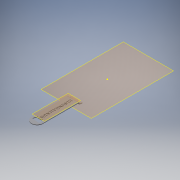
# Autodesk Inventor part: Rost_Heber
Saved by Autodesk Inventor 2018 (Build 220112000, 112)
## iProperties
Created: 2017-10-08
Part Number: Rost_Heber
Material: Generisch
Document SubType Name: Blech
Designer: Jan
Density: 1 g/cm^3
Sheet Metal Rule: Standard_mm
Appearance: Vorgabe
Flat Pattern Width: 4 cm
Flat Pattern Length: 16.3098 cm
Flat Pattern Area: 65.2391 cm^2
Sheet Metal Width: 40,000 mm
Sheet Metal Length: 163,098 mm
Sheet Metal Area: 6523,911 mm^2
Author: Jan
Autodesk Inventor part; units mm, degrees
ref_plane "YZ Plane" through (0, 0, 0) normal (1, 0, 0) x (0, 1, 0)
ref_plane "XZ Plane" through (0, 0, 0) normal (0, 1, 0) x (-1, 0, 0)
ref_plane "XY Plane" through (0, 0, 0) normal (0, 0, 1) x (1, 0, 0)
ref_plane "Arbeitsebene1" through (0, 0, 0) normal (0, 0, 1) x (1, 0, 0)
sketch "Skizze1" plane through (0, 0, 0) normal (0, 0, 1) x (1, 0, 0)
  arc A0 (31.5, -113.5) -> (26.5, -108.5) centre (26.5, -113.5) ccw
  line L0 (26.5, -108.5) -> (-26.5, -108.5)
  arc A1 (-26.5, -108.5) -> (-31.5, -113.5) centre (-26.5, -113.5) ccw
  line L1 (-31.5, -113.5) -> (-31.5, -124.5)
  line L2 (-31.5, -124.5) -> (-71, -124.5)
  arc A2 (-73, -122.5) -> (-71, -124.5) centre (-71, -122.5) ccw
  line L3 (-73, -122.5) -> (-73, 122.5)
  arc A3 (-71, 124.5) -> (-73, 122.5) centre (-71, 122.5) ccw
  line L4 (-71, 124.5) -> (71, 124.5)
  arc A4 (73, 122.5) -> (71, 124.5) centre (71, 122.5) ccw
  line L5 (73, 122.5) -> (73, -122.5)
  arc A5 (71, -124.5) -> (73, -122.5) centre (71, -122.5) ccw
  line L6 (71, -124.5) -> (31.5, -124.5)
  line L7 (31.5, -124.5) -> (31.5, -113.5)
  line L8 (-22.5, -122.5) -> (-22.5, -117.5)
  line L9 (-22.5, -117.5) -> (22.5, -117.5)
  line L10 (22.5, -117.5) -> (22.5, -122.5)
  line L11 (22.5, -122.5) -> (-22.5, -122.5)
  arc A6 (-81, -122.5) -> (-71, -132.5) centre (-71, -122.5) ccw
  line L12 (71, -132.5) -> (-71, -132.5)
  arc A7 (71, -132.5) -> (81, -122.5) centre (71, -122.5) ccw
  line L13 (81, 122.5) -> (81, -122.5)
  arc A8 (81, 122.5) -> (71, 132.5) centre (71, 122.5) ccw
  line L14 (-71, 132.5) -> (71, 132.5)
  arc A9 (-71, 132.5) -> (-81, 122.5) centre (-71, 122.5) ccw
  line L15 (-81, -122.5) -> (-81, 122.5)
  line L16 (-20, -118.5) -> (20, -118.5)
  line L17 (20, -118.5) -> (20, -248.5)
  line L18 (0, -268.5) -> (0, -268.5)
  line L19 (-20, -248.5) -> (-20, -118.5)
  line L20 (-116.2995, 0) -> (116.2995, 0)
  line L21 (0, -314.1009) -> (0, 209.3497)
  arc A10 (-20, -248.5) -> (0, -268.5) centre (0, -248.5) ccw
  arc A11 (0, -268.5) -> (20, -248.5) centre (0, -248.5) ccw
  point P0 (0, 0)
  dimension "HeberBreite" = 40
  dimension "d3" = 1
  dimension "HeberLänge" = 150
  dimension "d5" = 20
  measures "HeberBreite" distance of L16.start L16.end
  measures "d3" distance between parallel lines of L9 L16
  measures "HeberLänge" distance between parallel lines of L18 L16
  measures "d5" radius of A10
extrude "Grobblech1" add sketch "Skizze1" along normal blind 2 contours L21 L11 L19 L16 | L16 L17 L11 L21 | L21 L12 L19 L11 | L11 L17 L12 L21 | L21 A10 L19 L12 | L12 L17 A11 L21
sketch "Skizze2" plane through (20, -120.5, 2) normal (0, 1, 0) x (-1, 0, 0)
  line L0 (40, 0) -> (0, 0)
  line L1 (0, 0) -> (0, -8.05)
  line L2 (0, -8.05) -> (40, -8.05)
  line L3 (40, -8.05) -> (40, 0)
  constraints: 6 end point, 1 horizontal, 1 perpendicular, 1 vertical
edge flange "Lasche1" height 8.05 angle 90 thickness 2 bend radius 2 thickness toward (0, 1, 0) relief straight relief width 2 relief depth 1 edges at (0, -118.5, 0) wall of the first edge with corners at (-20, -120.5, 2) (20, -120.5, 2) (20, -120.5, -6.05) (-20, -120.5, -6.05)
bend "Biegung1"
corner "Ecke1"
sketch "Skizze3" plane through (-20, -120.5, -4.05) normal (0, 0, -1) x (-1, 0, 0)
  line L0 (-40, 0) -> (0, 0)
  line L1 (0, 0) -> (0, 12)
  line L2 (0, 12) -> (-40, 12)
  line L3 (-40, 12) -> (-40, 0)
  constraints: 6 end point, 1 horizontal, 1 perpendicular, 1 vertical
edge flange "Lasche2" height 12 angle 90 thickness 2 bend radius 2 thickness toward (0, 0, -1) relief straight relief width 2 relief depth 1 edges at (0, -118.5, -6.05) wall of the first edge with corners at (20, -120.5, -4.05) (-20, -120.5, -4.05) (-20, -108.5, -4.05) (20, -108.5, -4.05)
bend "Biegung2"
corner "Ecke2"
sketch "Skizze5" plane through (0, 0, 2) normal (0, 0, 1) x (1, 0, 0)
  line L0 (6.947, -239.8347) -> (6.947, -237.7708)
  arc A0 (10.3384, -238.5081) -> (6.947, -237.7708) centre (8.3903, -239.3005) ccw
  line L1 (10.3384, -238.5081) -> (13.6109, -248.7205)
  arc A1 (4.1757, -253.3868) -> (13.6109, -248.7205) centre (7.6304, -248.5) ccw
  line L2 (20, -122.5) -> (-20, -122.5) projected
  line L3 (-20, -248.5) -> (-20, -122.5) projected
  arc A2 (-20, -248.5) -> (20, -248.5) centre (0, -248.5) ccw projected
  line L4 (20, -122.5) -> (20, -248.5) projected
  line L5 (6.947, -239.8347) -> (-0.053, -239.8347)
  line L6 (4.1757, -253.3868) -> (-0.053, -253.3868)
  arc A3 (-7.053, -237.7708) -> (-10.3568, -238.3201) centre (-8.4962, -239.3005) ccw
  line L7 (-10.3568, -238.3201) -> (-13.7136, -248.7954)
  arc A4 (-13.7136, -248.7954) -> (-4.2816, -253.3868) centre (-7.7363, -248.5) ccw
  line L8 (-7.053, -239.8347) -> (-0.053, -239.8347)
  line L9 (-4.2816, -253.3868) -> (-0.053, -253.3868)
  line L10 (-7.053, -237.7708) -> (-7.053, -239.8347)
  line L11 (0, -312.7) -> (0, 206.7)
  dimension "d138" = 0
  constraints: 19 end point, 8 point on circle, 4 centre point, 3 parallel, 2 equal radius, 1 point on line, 1 vertical, 2 other
  measures "d138" vertical distance of A1.centre A2.centre
extrude "Ausklinkung1" cut sketch "Skizze5" against normal blind 2 contours L0 A0 L1 A1 L6 L11 L5 | L11 L6 L9 A4 L7 A3 L10 L8 L5
sketch "Skizze7" plane through (0, 0, 2) normal (0, 0, 1) x (1, 0, 0)
  point P0 (0, 0)
ref_plane "Arbeitsebene2" through (0, 0, 7) normal (0, 0, 1) x (1, 0, 0)
sketch "Skizze8" plane through (0, 0, 7) normal (0, 0, 1) x (1, 0, 0)
  line L0 (4.5218, -125.9558) -> (4.5218, -289.2753) construction
  line L1 (4.5218, -289.2753) -> (-6.6811, -289.2753) construction
  line L2 (-6.6811, -289.2753) -> (-6.6811, -125.9558) construction
  line L3 (-6.6811, -125.9558) -> (4.5218, -125.9558) construction
  line L4 (6.947, -239.8347) -> (6.947, -237.7708) projected
  arc A0 (10.3384, -238.5081) -> (6.947, -237.7708) centre (8.3903, -239.3005) ccw projected
  line L5 (10.3384, -238.5081) -> (13.6109, -248.7205) projected
  arc A1 (4.1757, -253.3868) -> (13.6109, -248.7205) centre (7.6304, -248.5) ccw projected
  line L6 (4.1757, -253.3868) -> (-4.2816, -253.3868) projected
  arc A2 (-13.7136, -248.7954) -> (-4.2816, -253.3868) centre (-7.7363, -248.5) ccw projected
  line L7 (-13.7136, -248.7954) -> (-10.3568, -238.3201) projected
  arc A3 (-7.053, -237.7708) -> (-10.3568, -238.3201) centre (-8.4962, -239.3005) ccw projected
  line L8 (-7.053, -237.7708) -> (-7.053, -239.8347) projected
  line L9 (-7.053, -239.8347) -> (6.947, -239.8347) projected
  line L10 (20, -122.5) -> (-20, -122.5) projected
  line L11 (-20, -248.5) -> (-20, -122.5) projected
  arc A4 (-20, -248.5) -> (20, -248.5) centre (0, -248.5) ccw projected
  line L12 (20, -122.5) -> (20, -248.5) projected
  line L13 (4.3421, -130.9167) -> (-4.6579, -130.9167)
  line L14 (-4.6579, -130.9167) -> (-4.6579, -127.4011)
  line L15 (-4.6579, -127.4011) -> (-4.6579, -127.198)
  spline S0 degree 2 poles (-4.6579, -127.198) (-4.6579, -126.9089) (-4.4782, -126.6042) (-4.3141, -126.6042) knots 0 0 0 1 2 2 2
  spline S1 degree 2 poles (-4.3141, -126.6042) (-4.0485, -126.6042) (-3.9626, -126.9167) knots 0 0 0 1 1 1
  spline S2 degree 2 poles (-3.9626, -126.9167) (-3.8844, -127.1824) (-3.8532, -127.2683) (-3.7907, -127.3152) knots 0 0 0 1 2 2 2
  spline S3 degree 2 poles (-3.7907, -127.3152) (-3.6891, -127.4089) (-3.4548, -127.4089) knots 0 0 0 1 1 1
  line L16 (-3.4548, -127.4089) -> (3.139, -127.4089)
  spline S4 degree 2 poles (3.139, -127.4089) (3.3734, -127.4089) (3.4749, -127.3152) knots 0 0 0 1 1 1
  spline S5 degree 2 poles (3.4749, -127.3152) (3.5374, -127.2683) (3.5687, -127.1824) (3.639, -126.9167) knots 0 0 0 1 2 2 2
  spline S6 degree 2 poles (3.639, -126.9167) (3.7249, -126.6042) (3.9984, -126.6042) knots 0 0 0 1 1 1
  spline S7 degree 2 poles (3.9984, -126.6042) (4.1624, -126.6042) (4.3421, -126.9089) (4.3421, -127.198) knots 0 0 0 1 2 2 2
  line L17 (4.3421, -127.198) -> (4.3421, -127.4011)
  line L18 (4.3421, -127.4011) -> (4.3421, -130.9167)
  line L19 (-4.6579, -131.6355) -> (-3.9469, -131.6355)
  spline S8 degree 2 poles (-3.9469, -131.6355) (-3.8844, -132.1511) (-3.6423, -132.823) (-3.4001, -133.1589) knots 0 0 0 1 2 2 2
  spline S9 degree 2 poles (-3.4001, -133.1589) (-3.1579, -133.5027) (-2.6344, -133.9011) (-2.2048, -134.0886) knots 0 0 0 1 2 2 2
  spline S10 degree 2 poles (-2.2048, -134.0886) (-1.9938, -134.1746) (-1.8454, -134.3621) (-1.8454, -134.5261) knots 0 0 0 1 2 2 2
  spline S11 degree 2 poles (-1.8454, -134.5261) (-1.8454, -134.7527) (-2.0641, -134.9246) (-2.3298, -134.9246) knots 0 0 0 1 2 2 2
  line L20 (-2.3298, -134.9246) -> (-4.6579, -134.9246)
  line L21 (-4.6579, -134.9246) -> (-4.6579, -131.6355)
  line L22 (4.3421, -131.6277) -> (4.3421, -134.8152)
  line L23 (4.3421, -134.8152) -> (2.0062, -134.8152)
  spline S12 degree 2 poles (2.0062, -134.8152) (1.8031, -134.8152) (1.6234, -134.6277) (1.6234, -134.4167) knots 0 0 0 1 2 2 2
  spline S13 degree 2 poles (1.6234, -134.4167) (1.6234, -134.2449) (1.7406, -134.0886) (1.9281, -134.0183) knots 0 0 0 1 2 2 2
  spline S14 degree 2 poles (1.9281, -134.0183) (2.6859, -133.7136) (3.4906, -132.5496) (3.5687, -131.6277) knots 0 0 0 1 2 2 2
  line L24 (3.5687, -131.6277) -> (4.3421, -131.6277)
  line L25 (-0.4626, -131.5886) -> (0.3031, -131.5886)
  spline S15 degree 2 poles (0.3031, -131.5886) (0.4906, -132.0496) (0.9281, -132.4871) (1.2874, -132.5964) knots 0 0 0 1 2 2 2
  spline S16 degree 2 poles (1.2874, -132.5964) (1.5374, -132.6589) (1.7327, -132.8621) (1.7327, -133.0496) knots 0 0 0 1 2 2 2
  spline S17 degree 2 poles (1.7327, -133.0496) (1.7327, -133.3074) (1.5687, -133.4011) knots 0 0 0 1 1 1
  spline S18 degree 2 poles (1.5687, -133.4011) (1.4827, -133.4558) (1.1781, -133.4558) knots 0 0 0 1 1 1
  line L26 (1.1781, -133.4558) -> (-1.3376, -133.4558)
  spline S19 degree 2 poles (-1.3376, -133.4558) (-1.6501, -133.4558) (-1.8844, -133.2917) (-1.8844, -133.0652) knots 0 0 0 1 2 2 2
  spline S20 degree 2 poles (-1.8844, -133.0652) (-1.8844, -132.8855) (-1.6969, -132.6824) (-1.4782, -132.6199) knots 0 0 0 1 2 2 2
  spline S21 degree 2 poles (-1.4782, -132.6199) (-1.0251, -132.4792) (-0.5407, -131.9871) (-0.4626, -131.5886) knots 0 0 0 1 2 2 2
  line L27 (-4.6579, -140.4324) -> (-4.6579, -136.9089)
  line L28 (-4.6579, -136.9089) -> (-4.6579, -136.7058)
  spline S22 degree 2 poles (-4.6579, -136.7058) (-4.6579, -136.4167) (-4.4782, -136.1121) (-4.3141, -136.1121) knots 0 0 0 1 2 2 2
  spline S23 degree 2 poles (-4.3141, -136.1121) (-4.0485, -136.1121) (-3.9626, -136.4246) knots 0 0 0 1 1 1
  spline S24 degree 2 poles (-3.9626, -136.4246) (-3.8844, -136.6902) (-3.8532, -136.7761) (-3.7907, -136.823) knots 0 0 0 1 2 2 2
  spline S25 degree 2 poles (-3.7907, -136.823) (-3.6891, -136.9167) (-3.4548, -136.9167) knots 0 0 0 1 1 1
  line L29 (-3.4548, -136.9167) -> (3.139, -136.9167)
  spline S26 degree 2 poles (3.139, -136.9167) (3.3734, -136.9167) (3.4749, -136.823) knots 0 0 0 1 1 1
  spline S27 degree 2 poles (3.4749, -136.823) (3.5374, -136.7761) (3.5687, -136.6902) (3.639, -136.4246) knots 0 0 0 1 2 2 2
  spline S28 degree 2 poles (3.639, -136.4246) (3.7249, -136.1121) (3.9984, -136.1121) knots 0 0 0 1 1 1
  spline S29 degree 2 poles (3.9984, -136.1121) (4.1624, -136.1121) (4.3421, -136.4167) (4.3421, -136.7058) knots 0 0 0 1 2 2 2
  line L30 (4.3421, -136.7058) -> (4.3421, -136.9089)
  line L31 (4.3421, -136.9089) -> (4.3421, -140.4324)
  line L32 (4.3421, -140.4324) -> (4.3421, -140.6355)
  spline S30 degree 2 poles (4.3421, -140.6355) (4.3421, -140.9246) (4.1624, -141.2292) (3.9984, -141.2292) knots 0 0 0 1 2 2 2
  spline S31 degree 2 poles (3.9984, -141.2292) (3.7249, -141.2292) (3.639, -140.9167) knots 0 0 0 1 1 1
  spline S32 degree 2 poles (3.639, -140.9167) (3.5687, -140.6511) (3.5374, -140.5652) (3.4749, -140.5183) knots 0 0 0 1 2 2 2
  spline S33 degree 2 poles (3.4749, -140.5183) (3.3734, -140.4246) (3.139, -140.4246) knots 0 0 0 1 1 1
  line L33 (3.139, -140.4246) -> (-3.4548, -140.4246)
  spline S34 degree 2 poles (-3.4548, -140.4246) (-3.6891, -140.4246) (-3.7907, -140.5183) knots 0 0 0 1 1 1
  spline S35 degree 2 poles (-3.7907, -140.5183) (-3.8532, -140.5652) (-3.8844, -140.6511) (-3.9626, -140.9167) knots 0 0 0 1 2 2 2
  spline S36 degree 2 poles (-3.9626, -140.9167) (-4.0485, -141.2292) (-4.3141, -141.2292) knots 0 0 0 1 1 1
  spline S37 degree 2 poles (-4.3141, -141.2292) (-4.4782, -141.2292) (-4.6579, -140.9246) (-4.6579, -140.6355) knots 0 0 0 1 2 2 2
  line L34 (-4.6579, -140.6355) -> (-4.6579, -140.4324)
  line L35 (4.5218, -146.1824) -> (3.764, -146.1824)
  spline S38 degree 2 poles (3.764, -146.1824) (3.6468, -145.6902) (3.1781, -145.1746) (2.8421, -145.1746) knots 0 0 0 1 2 2 2
  spline S39 degree 2 poles (2.8421, -145.1746) (2.5062, -145.1746) (2.014, -145.6042) (1.7874, -146.0808) knots 0 0 0 1 2 2 2
  spline S40 degree 2 poles (1.7874, -146.0808) (1.639, -146.4167) (1.2093, -147.5886) knots 0 0 0 1 1 1
  spline S41 degree 2 poles (1.2093, -147.5886) (0.9515, -148.2996) (0.5374, -149.0808) (0.2249, -149.4324) knots 0 0 0 1 2 2 2
  spline S42 degree 2 poles (0.2249, -149.4324) (-0.5876, -150.3621) (-1.7204, -150.3621) knots 0 0 0 1 1 1
  spline S43 degree 2 poles (-1.7204, -150.3621) (-2.5641, -150.3621) (-3.9782, -149.3464) (-4.3844, -148.4636) knots 0 0 0 1 2 2 2
  spline S44 degree 2 poles (-4.3844, -148.4636) (-4.5954, -147.9871) (-4.8376, -146.8621) (-4.8376, -146.3699) knots 0 0 0 1 2 2 2
  line L36 (-4.8376, -146.3699) -> (-4.0876, -146.3699)
  spline S45 degree 2 poles (-4.0876, -146.3699) (-3.9469, -147.0574) (-3.4548, -147.6667) (-3.0329, -147.6667) knots 0 0 0 1 2 2 2
  spline S46 degree 2 poles (-3.0329, -147.6667) (-2.5876, -147.6667) (-2.2516, -147.1902) knots 0 0 0 1 1 1
  spline S47 degree 2 poles (-2.2516, -147.1902) (-2.0329, -146.8777) (-1.7126, -145.9871) knots 0 0 0 1 1 1
  spline S48 degree 2 poles (-1.7126, -145.9871) (-1.3532, -145.0183) (-1.0485, -144.2996) (-0.8454, -143.9636) knots 0 0 0 1 2 2 2
  spline S49 degree 2 poles (-0.8454, -143.9636) (0.0374, -142.4792) (1.5062, -142.4792) knots 0 0 0 1 1 1
  spline S50 degree 2 poles (1.5062, -142.4792) (2.2562, -142.4792) (3.5296, -143.2214) (3.9202, -143.8855) knots 0 0 0 1 2 2 2
  spline S51 degree 2 poles (3.9202, -143.8855) (4.4593, -144.8152) (4.5218, -146.1824) knots 0 0 0 1 1 1
  line L37 (-4.0876, -145.7683) -> (-4.8376, -145.7683)
  spline S52 degree 2 poles (-4.8376, -145.7683) (-4.8376, -145.1199) (-4.5329, -144.3386) knots 0 0 0 1 1 1
  spline S53 degree 2 poles (-4.5329, -144.3386) (-4.4157, -144.0417) (-4.3532, -143.823) (-4.3532, -143.7214) knots 0 0 0 1 2 2 2
  spline S54 degree 2 poles (-4.3532, -143.7214) (-4.3532, -143.5652) (-4.4391, -143.4011) (-4.611, -143.2292) knots 0 0 0 1 2 2 2
  spline S55 degree 2 poles (-4.611, -143.2292) (-4.7516, -143.0886) (-4.7516, -142.9246) knots 0 0 0 1 1 1
  spline S56 degree 2 poles (-4.7516, -142.9246) (-4.7516, -142.4792) (-4.1813, -142.4792) knots 0 0 0 1 1 1
  line L38 (-4.1813, -142.4792) -> (-1.7829, -142.4792)
  spline S57 degree 2 poles (-1.7829, -142.4792) (-1.6032, -142.4792) (-1.3454, -142.7292) (-1.3376, -142.9246) knots 0 0 0 1 2 2 2
  spline S58 degree 2 poles (-1.3376, -142.9246) (-1.3298, -143.0964) (-1.5094, -143.2917) (-1.736, -143.3621) knots 0 0 0 1 2 2 2
  spline S59 degree 2 poles (-1.736, -143.3621) (-2.2985, -143.5496) (-3.2907, -144.2371) (-3.6266, -144.6902) knots 0 0 0 1 2 2 2
  spline S60 degree 2 poles (-3.6266, -144.6902) (-3.986, -145.1589) (-4.0876, -145.7683) knots 0 0 0 1 1 1
  line L39 (3.764, -146.8074) -> (4.4906, -146.8074)
  spline S61 degree 2 poles (4.4906, -146.8074) (4.4593, -147.2839) (4.3031, -147.9792) (4.0765, -148.6199) knots 0 0 0 1 2 2 2
  spline S62 degree 2 poles (4.0765, -148.6199) (4.0218, -148.7761) (4.0218, -148.8777) knots 0 0 0 1 1 1
  spline S63 degree 2 poles (4.0218, -148.8777) (4.0218, -149.0261) (4.1077, -149.1042) knots 0 0 0 1 1 1
  line L40 (4.1077, -149.1042) -> (4.3031, -149.2761)
  spline S64 degree 2 poles (4.3031, -149.2761) (4.4515, -149.4011) (4.4515, -149.5808) knots 0 0 0 1 1 1
  spline S65 degree 2 poles (4.4515, -149.5808) (4.4515, -149.7996) (4.1937, -149.9949) (3.9202, -149.9949) knots 0 0 0 1 2 2 2
  line L41 (3.9202, -149.9949) -> (1.7406, -149.9949)
  spline S66 degree 2 poles (1.7406, -149.9949) (1.5452, -149.9949) (1.3031, -149.7371) (1.3031, -149.5261) knots 0 0 0 1 2 2 2
  spline S67 degree 2 poles (1.3031, -149.5261) (1.3031, -149.3699) (1.389, -149.2371) knots 0 0 0 1 1 1
  spline S68 degree 2 poles (1.389, -149.2371) (1.4437, -149.1667) (1.5921, -149.0808) (1.7718, -149.0417) knots 0 0 0 1 2 2 2
  spline S69 degree 2 poles (1.7718, -149.0417) (2.0999, -148.948) (2.7796, -148.5261) (3.0531, -148.2371) knots 0 0 0 1 2 2 2
  spline S70 degree 2 poles (3.0531, -148.2371) (3.5921, -147.6667) (3.764, -146.8074) knots 0 0 0 1 1 1
  line L42 (4.3421, -155.9167) -> (-4.6579, -155.9167)
  line L43 (-4.6579, -155.9167) -> (-4.6579, -152.4011)
  line L44 (-4.6579, -152.4011) -> (-4.6579, -152.198)
  spline S71 degree 2 poles (-4.6579, -152.198) (-4.6579, -151.9089) (-4.4782, -151.6042) (-4.3141, -151.6042) knots 0 0 0 1 2 2 2
  spline S72 degree 2 poles (-4.3141, -151.6042) (-4.0485, -151.6042) (-3.9626, -151.9167) knots 0 0 0 1 1 1
  spline S73 degree 2 poles (-3.9626, -151.9167) (-3.8844, -152.1824) (-3.8532, -152.2683) (-3.7907, -152.3152) knots 0 0 0 1 2 2 2
  spline S74 degree 2 poles (-3.7907, -152.3152) (-3.6891, -152.4089) (-3.4548, -152.4089) knots 0 0 0 1 1 1
  line L45 (-3.4548, -152.4089) -> (3.139, -152.4089)
  spline S75 degree 2 poles (3.139, -152.4089) (3.3734, -152.4089) (3.4749, -152.3152) knots 0 0 0 1 1 1
  spline S76 degree 2 poles (3.4749, -152.3152) (3.5374, -152.2683) (3.5687, -152.1824) (3.639, -151.9167) knots 0 0 0 1 2 2 2
  spline S77 degree 2 poles (3.639, -151.9167) (3.7249, -151.6042) (3.9984, -151.6042) knots 0 0 0 1 1 1
  spline S78 degree 2 poles (3.9984, -151.6042) (4.1624, -151.6042) (4.3421, -151.9089) (4.3421, -152.198) knots 0 0 0 1 2 2 2
  line L46 (4.3421, -152.198) -> (4.3421, -152.4011)
  line L47 (4.3421, -152.4011) -> (4.3421, -155.9167)
  line L48 (-4.6579, -156.6355) -> (-3.9469, -156.6355)
  spline S79 degree 2 poles (-3.9469, -156.6355) (-3.8844, -157.1511) (-3.6423, -157.823) (-3.4001, -158.1589) knots 0 0 0 1 2 2 2
  spline S80 degree 2 poles (-3.4001, -158.1589) (-3.1579, -158.5027) (-2.6344, -158.9011) (-2.2048, -159.0886) knots 0 0 0 1 2 2 2
  spline S81 degree 2 poles (-2.2048, -159.0886) (-1.9938, -159.1746) (-1.8454, -159.3621) (-1.8454, -159.5261) knots 0 0 0 1 2 2 2
  spline S82 degree 2 poles (-1.8454, -159.5261) (-1.8454, -159.7527) (-2.0641, -159.9246) (-2.3298, -159.9246) knots 0 0 0 1 2 2 2
  line L49 (-2.3298, -159.9246) -> (-4.6579, -159.9246)
  line L50 (-4.6579, -159.9246) -> (-4.6579, -156.6355)
  line L51 (4.3421, -156.6277) -> (4.3421, -159.8152)
  line L52 (4.3421, -159.8152) -> (2.0062, -159.8152)
  spline S83 degree 2 poles (2.0062, -159.8152) (1.8031, -159.8152) (1.6234, -159.6277) (1.6234, -159.4167) knots 0 0 0 1 2 2 2
  spline S84 degree 2 poles (1.6234, -159.4167) (1.6234, -159.2449) (1.7406, -159.0886) (1.9281, -159.0183) knots 0 0 0 1 2 2 2
  spline S85 degree 2 poles (1.9281, -159.0183) (2.6859, -158.7136) (3.4906, -157.5496) (3.5687, -156.6277) knots 0 0 0 1 2 2 2
  line L53 (3.5687, -156.6277) -> (4.3421, -156.6277)
  line L54 (-0.4626, -156.5886) -> (0.3031, -156.5886)
  spline S86 degree 2 poles (0.3031, -156.5886) (0.4906, -157.0496) (0.9281, -157.4871) (1.2874, -157.5964) knots 0 0 0 1 2 2 2
  spline S87 degree 2 poles (1.2874, -157.5964) (1.5374, -157.6589) (1.7327, -157.8621) (1.7327, -158.0496) knots 0 0 0 1 2 2 2
  spline S88 degree 2 poles (1.7327, -158.0496) (1.7327, -158.3074) (1.5687, -158.4011) knots 0 0 0 1 1 1
  spline S89 degree 2 poles (1.5687, -158.4011) (1.4827, -158.4558) (1.1781, -158.4558) knots 0 0 0 1 1 1
  line L55 (1.1781, -158.4558) -> (-1.3376, -158.4558)
  spline S90 degree 2 poles (-1.3376, -158.4558) (-1.6501, -158.4558) (-1.8844, -158.2917) (-1.8844, -158.0652) knots 0 0 0 1 2 2 2
  spline S91 degree 2 poles (-1.8844, -158.0652) (-1.8844, -157.8855) (-1.6969, -157.6824) (-1.4782, -157.6199) knots 0 0 0 1 2 2 2
  spline S92 degree 2 poles (-1.4782, -157.6199) (-1.0251, -157.4792) (-0.5407, -156.9871) (-0.4626, -156.5886) knots 0 0 0 1 2 2 2
  line L56 (4.3421, -165.5886) -> (-1.7516, -169.7917)
  line L57 (-1.7516, -169.7917) -> (-4.6579, -169.7917)
  line L58 (-4.6579, -169.7917) -> (-4.6579, -167.6355)
  line L59 (-4.6579, -167.6355) -> (3.0531, -162.2683)
  spline S93 degree 2 poles (3.0531, -162.2683) (3.3109, -162.0886) (3.5062, -161.8699) (3.5531, -161.698) knots 0 0 0 1 2 2 2
  line L60 (3.5531, -161.698) -> (3.6468, -161.3933)
  spline S94 degree 2 poles (3.6468, -161.3933) (3.6781, -161.2761) (3.8499, -161.1355) (3.9515, -161.1355) knots 0 0 0 1 2 2 2
  spline S95 degree 2 poles (3.9515, -161.1355) (4.0687, -161.1355) (4.2562, -161.2761) (4.2952, -161.3933) knots 0 0 0 1 2 2 2
  spline S96 degree 2 poles (4.2952, -161.3933) (4.3421, -161.5261) (4.3421, -162.1199) knots 0 0 0 1 1 1
  line L61 (4.3421, -162.1199) -> (4.3421, -165.5886)
  line L62 (2.0218, -162.2761) -> (0.8656, -163.1121)
  line L63 (0.8656, -163.1121) -> (-2.6657, -163.1121)
  spline S97 degree 2 poles (-2.6657, -163.1121) (-3.1266, -163.1121) (-3.7204, -163.4871) (-3.9157, -163.8855) knots 0 0 0 1 2 2 2
  line L64 (-3.9157, -163.8855) -> (-4.0251, -164.1277)
  spline S98 degree 2 poles (-4.0251, -164.1277) (-4.1266, -164.3308) (-4.3219, -164.3308) knots 0 0 0 1 1 1
  spline S99 degree 2 poles (-4.3219, -164.3308) (-4.4704, -164.3308) (-4.5719, -164.1824) knots 0 0 0 1 1 1
  spline S100 degree 2 poles (-4.5719, -164.1824) (-4.6579, -164.0574) (-4.6579, -163.6589) knots 0 0 0 1 1 1
  line L65 (-4.6579, -163.6589) -> (-4.6579, -161.8308)
  spline S101 degree 2 poles (-4.6579, -161.8308) (-4.6579, -161.1121) (-4.3141, -161.1121) knots 0 0 0 1 1 1
  spline S102 degree 2 poles (-4.3141, -161.1121) (-4.1969, -161.1121) (-4.0563, -161.2605) (-3.9391, -161.5183) knots 0 0 0 1 2 2 2
  spline S103 degree 2 poles (-3.9391, -161.5183) (-3.5876, -162.2761) (-2.6657, -162.2761) knots 0 0 0 1 1 1
  line L66 (-2.6657, -162.2761) -> (2.0218, -162.2761)
  line L67 (-0.6969, -169.7917) -> (0.4827, -168.9558)
  line L68 (0.4827, -168.9558) -> (2.3109, -168.9558)
  spline S104 degree 2 poles (2.3109, -168.9558) (2.8656, -168.9558) (3.4515, -168.5652) (3.6624, -168.0808) knots 0 0 0 1 2 2 2
  spline S105 degree 2 poles (3.6624, -168.0808) (3.7249, -167.9089) (3.8812, -167.7839) (3.9984, -167.7839) knots 0 0 0 1 2 2 2
  spline S106 degree 2 poles (3.9984, -167.7839) (4.1781, -167.7839) (4.3421, -168.0652) (4.3421, -168.3699) knots 0 0 0 1 2 2 2
  line L69 (4.3421, -168.3699) -> (4.3421, -170.3464)
  spline S107 degree 2 poles (4.3421, -170.3464) (4.3421, -170.7527) (4.2327, -170.8777) knots 0 0 0 1 1 1
  spline S108 degree 2 poles (4.2327, -170.8777) (4.1312, -171.0105) (3.9827, -171.0105) knots 0 0 0 1 1 1
  spline S109 degree 2 poles (3.9827, -171.0105) (3.8499, -171.0105) (3.7093, -170.8621) (3.5921, -170.573) knots 0 0 0 1 2 2 2
  spline S110 degree 2 poles (3.5921, -170.573) (3.4124, -170.1589) (3.0452, -169.9402) knots 0 0 0 1 1 1
  spline S111 degree 2 poles (3.0452, -169.9402) (2.7718, -169.7917) (2.3109, -169.7917) knots 0 0 0 1 1 1
  line L70 (2.3109, -169.7917) -> (-0.6969, -169.7917)
  line L71 (4.3421, -176.2996) -> (-4.6579, -176.2996)
  line L72 (-4.6579, -176.2996) -> (-4.6579, -172.7839)
  line L73 (-4.6579, -172.7839) -> (-4.6579, -172.5808)
  spline S112 degree 2 poles (-4.6579, -172.5808) (-4.6579, -172.2917) (-4.4782, -171.9871) (-4.3141, -171.9871) knots 0 0 0 1 2 2 2
  spline S113 degree 2 poles (-4.3141, -171.9871) (-4.0485, -171.9871) (-3.9626, -172.2996) knots 0 0 0 1 1 1
  spline S114 degree 2 poles (-3.9626, -172.2996) (-3.8844, -172.5652) (-3.8532, -172.6511) (-3.7907, -172.698) knots 0 0 0 1 2 2 2
  spline S115 degree 2 poles (-3.7907, -172.698) (-3.6891, -172.7917) (-3.4548, -172.7917) knots 0 0 0 1 1 1
  line L74 (-3.4548, -172.7917) -> (3.139, -172.7917)
  spline S116 degree 2 poles (3.139, -172.7917) (3.3734, -172.7917) (3.4749, -172.698) knots 0 0 0 1 1 1
  spline S117 degree 2 poles (3.4749, -172.698) (3.5374, -172.6511) (3.5687, -172.5652) (3.639, -172.2996) knots 0 0 0 1 2 2 2
  spline S118 degree 2 poles (3.639, -172.2996) (3.7249, -171.9871) (3.9984, -171.9871) knots 0 0 0 1 1 1
  spline S119 degree 2 poles (3.9984, -171.9871) (4.1624, -171.9871) (4.3421, -172.2917) (4.3421, -172.5808) knots 0 0 0 1 2 2 2
  line L75 (4.3421, -172.5808) -> (4.3421, -172.7839)
  line L76 (4.3421, -172.7839) -> (4.3421, -176.2996)
  spline S120 degree 2 poles (-0.0016, -178.7605) (-0.1188, -179.4714) (-0.3376, -180.2449) (-0.5094, -180.5496) knots 0 0 0 1 2 2 2
  spline S121 degree 2 poles (-0.5094, -180.5496) (-0.7985, -181.0808) (-1.7282, -181.6433) (-2.2985, -181.6433) knots 0 0 0 1 2 2 2
  spline S122 degree 2 poles (-2.2985, -181.6433) (-3.4235, -181.6433) (-4.0563, -180.6433) knots 0 0 0 1 1 1
  spline S123 degree 2 poles (-4.0563, -180.6433) (-4.3844, -180.1355) (-4.6579, -178.8933) (-4.6579, -177.8855) knots 0 0 0 1 2 2 2
  line L77 (-4.6579, -177.8855) -> (-4.6579, -176.9402)
  line L78 (-4.6579, -176.9402) -> (-3.9626, -176.9402)
  spline S124 degree 2 poles (-3.9626, -176.9402) (-3.9469, -177.2605) (-3.8376, -177.6199) (-3.7048, -177.7683) knots 0 0 0 1 2 2 2
  spline S125 degree 2 poles (-3.7048, -177.7683) (-3.4548, -178.0261) (-2.9469, -178.0261) knots 0 0 0 1 1 1
  line L79 (-2.9469, -178.0261) -> (-1.4469, -178.0261)
  spline S126 degree 2 poles (-1.4469, -178.0261) (-1.1188, -178.0261) (-0.7516, -177.8933) (-0.5954, -177.7136) knots 0 0 0 1 2 2 2
  spline S127 degree 2 poles (-0.5954, -177.7136) (-0.4782, -177.5808) (-0.3766, -177.2605) (-0.3376, -176.9714) knots 0 0 0 1 2 2 2
  line L80 (-0.3376, -176.9714) -> (0.3421, -176.9714)
  spline S128 degree 2 poles (0.3421, -176.9714) (0.3656, -177.2605) (0.4593, -177.5886) (0.5609, -177.7214) knots 0 0 0 1 2 2 2
  spline S129 degree 2 poles (0.5609, -177.7214) (0.6624, -177.8464) (0.9749, -178.0183) (1.1077, -178.0261) knots 0 0 0 1 2 2 2
  line L81 (1.1077, -178.0261) -> (1.4749, -178.0261)
  line L82 (1.4749, -178.0261) -> (2.6156, -178.0261)
  spline S130 degree 2 poles (2.6156, -178.0261) (2.7952, -178.0261) (3.1859, -177.8855) (3.2952, -177.7839) knots 0 0 0 1 2 2 2
  spline S131 degree 2 poles (3.2952, -177.7839) (3.4437, -177.6277) (3.5921, -177.2605) (3.6156, -176.9402) knots 0 0 0 1 2 2 2
  line L83 (3.6156, -176.9402) -> (4.3421, -176.9402)
  line L84 (4.3421, -176.9402) -> (4.3421, -177.8542)
  spline S132 degree 2 poles (4.3421, -177.8542) (4.3421, -179.6589) (3.7249, -180.6042) knots 0 0 0 1 1 1
  spline S133 degree 2 poles (3.7249, -180.6042) (3.4359, -181.0417) (2.6312, -181.5027) (2.1624, -181.5027) knots 0 0 0 1 2 2 2
  spline S134 degree 2 poles (2.1624, -181.5027) (1.7015, -181.5027) (0.889, -181.0339) (0.6156, -180.6121) knots 0 0 0 1 2 2 2
  spline S135 degree 2 poles (0.6156, -180.6121) (0.4046, -180.3074) (0.139, -179.5027) (-0.0016, -178.7605) knots 0 0 0 1 2 2 2
  line L85 (4.3421, -186.0027) -> (4.3421, -189.1902)
  line L86 (4.3421, -189.1902) -> (-3.4079, -191.3855)
  spline S136 degree 2 poles (-3.4079, -191.3855) (-3.611, -191.448) (-3.7673, -191.5261) knots 0 0 0 1 1 1
  spline S137 degree 2 poles (-3.7673, -191.5261) (-3.8923, -191.5964) (-3.9704, -191.8464) knots 0 0 0 1 1 1
  spline S138 degree 2 poles (-3.9704, -191.8464) (-4.0485, -192.0496) (-4.1891, -192.2058) (-4.3141, -192.2058) knots 0 0 0 1 2 2 2
  spline S139 degree 2 poles (-4.3141, -192.2058) (-4.6579, -192.2058) (-4.6579, -191.5964) knots 0 0 0 1 1 1
  line L87 (-4.6579, -191.5964) -> (-4.6579, -187.6433)
  spline S140 degree 2 poles (-4.6579, -187.6433) (-4.6579, -187.4089) (-4.4626, -187.1277) (-4.3063, -187.1277) knots 0 0 0 1 2 2 2
  spline S141 degree 2 poles (-4.3063, -187.1277) (-4.1735, -187.1277) (-4.0407, -187.2527) (-3.9469, -187.4792) knots 0 0 0 1 2 2 2
  spline S142 degree 2 poles (-3.9469, -187.4792) (-3.8766, -187.6355) (-3.7204, -187.7605) (-3.6032, -187.7605) knots 0 0 0 1 2 2 2
  spline S143 degree 2 poles (-3.6032, -187.7605) (-3.486, -187.7605) (-3.4001, -187.7371) knots 0 0 0 1 1 1
  line L88 (-3.4001, -187.7371) -> (-2.4469, -187.4792)
  line L89 (-2.4469, -187.4792) -> (-2.4469, -185.2761)
  line L90 (-2.4469, -185.2761) -> (-1.6657, -185.4871)
  line L91 (-1.6657, -185.4871) -> (-1.6657, -187.2605)
  line L92 (-1.6657, -187.2605) -> (3.6937, -185.8074)
  line L93 (3.6937, -185.8074) -> (4.3421, -186.0027)
  line L94 (2.6624, -185.4558) -> (1.3031, -185.8621)
  line L95 (1.3031, -185.8621) -> (-2.9548, -184.4558)
  spline S144 degree 2 poles (-2.9548, -184.4558) (-3.1423, -184.3933) (-3.2985, -184.3933) knots 0 0 0 1 1 1
  spline S145 degree 2 poles (-3.2985, -184.3933) (-3.7126, -184.3933) (-3.8923, -184.8621) knots 0 0 0 1 1 1
  line L96 (-3.8923, -184.8621) -> (-4.0016, -185.1355)
  spline S146 degree 2 poles (-4.0016, -185.1355) (-4.0954, -185.4011) (-4.3298, -185.4011) knots 0 0 0 1 1 1
  spline S147 degree 2 poles (-4.3298, -185.4011) (-4.6579, -185.4011) (-4.6579, -184.823) knots 0 0 0 1 1 1
  line L97 (-4.6579, -184.823) -> (-4.6579, -182.8152)
  spline S148 degree 2 poles (-4.6579, -182.8152) (-4.6579, -182.5261) (-4.4548, -182.1824) (-4.2751, -182.1824) knots 0 0 0 1 2 2 2
  spline S149 degree 2 poles (-4.2751, -182.1824) (-4.0876, -182.1824) (-3.9626, -182.5339) knots 0 0 0 1 1 1
  spline S150 degree 2 poles (-3.9626, -182.5339) (-3.8376, -182.8542) (-3.6501, -183.1667) (-3.486, -183.3074) knots 0 0 0 1 2 2 2
  spline S151 degree 2 poles (-3.486, -183.3074) (-3.2126, -183.5261) (-2.7673, -183.6667) knots 0 0 0 1 1 1
  line L98 (-2.7673, -183.6667) -> (2.6624, -185.4558)
  line L99 (0.264, -198.0183) -> (0.264, -199.3074)
  line L100 (0.264, -199.3074) -> (3.139, -199.3074)
  spline S152 degree 2 poles (3.139, -199.3074) (3.514, -199.3074) (3.5765, -199.0808) knots 0 0 0 1 1 1
  line L101 (3.5765, -199.0808) -> (3.639, -198.823)
  spline S153 degree 2 poles (3.639, -198.823) (3.7249, -198.5261) (3.9984, -198.5261) knots 0 0 0 1 1 1
  spline S154 degree 2 poles (3.9984, -198.5261) (4.3421, -198.5261) (4.3421, -199.0964) knots 0 0 0 1 1 1
  line L102 (4.3421, -199.0964) -> (4.3421, -199.2996)
  line L103 (4.3421, -199.2996) -> (4.3421, -202.8152)
  line L104 (4.3421, -202.8152) -> (4.3421, -203.0261)
  spline S155 degree 2 poles (4.3421, -203.0261) (4.3421, -203.6199) (3.9984, -203.6199) knots 0 0 0 1 1 1
  spline S156 degree 2 poles (3.9984, -203.6199) (3.7249, -203.6199) (3.639, -203.3074) knots 0 0 0 1 1 1
  spline S157 degree 2 poles (3.639, -203.3074) (3.5687, -203.0417) (3.5374, -202.9558) (3.4749, -202.9089) knots 0 0 0 1 2 2 2
  spline S158 degree 2 poles (3.4749, -202.9089) (3.3734, -202.8152) (3.139, -202.8152) knots 0 0 0 1 1 1
  line L105 (3.139, -202.8152) -> (-3.4313, -202.8152)
  spline S159 degree 2 poles (-3.4313, -202.8152) (-3.7985, -202.8152) (-3.8766, -203.0496) knots 0 0 0 1 1 1
  line L106 (-3.8766, -203.0496) -> (-3.9469, -203.3074)
  spline S160 degree 2 poles (-3.9469, -203.3074) (-4.0329, -203.6199) (-4.3063, -203.6199) knots 0 0 0 1 1 1
  spline S161 degree 2 poles (-4.3063, -203.6199) (-4.6579, -203.6199) (-4.6579, -203.0261) knots 0 0 0 1 1 1
  line L107 (-4.6579, -203.0261) -> (-4.6579, -202.8152)
  line L108 (-4.6579, -202.8152) -> (-4.6579, -199.2996)
  line L109 (-4.6579, -199.2996) -> (-4.6579, -199.0808)
  spline S162 degree 2 poles (-4.6579, -199.0808) (-4.6579, -198.5261) (-4.3063, -198.5261) knots 0 0 0 1 1 1
  spline S163 degree 2 poles (-4.3063, -198.5261) (-4.0329, -198.5261) (-3.9469, -198.823) knots 0 0 0 1 1 1
  line L110 (-3.9469, -198.823) -> (-3.8766, -199.0808)
  spline S164 degree 2 poles (-3.8766, -199.0808) (-3.8141, -199.3074) (-3.4313, -199.3074) knots 0 0 0 1 1 1
  line L111 (-3.4313, -199.3074) -> (-0.3923, -199.3074)
  line L112 (-0.3923, -199.3074) -> (-0.3923, -198.0183)
  line L113 (-0.3923, -198.0183) -> (0.264, -198.0183)
  line L114 (-4.6579, -197.3542) -> (-4.6579, -193.8308)
  line L115 (-4.6579, -193.8308) -> (-4.6579, -193.6277)
  spline S165 degree 2 poles (-4.6579, -193.6277) (-4.6579, -193.3386) (-4.4782, -193.0339) (-4.3141, -193.0339) knots 0 0 0 1 2 2 2
  spline S166 degree 2 poles (-4.3141, -193.0339) (-4.0485, -193.0339) (-3.9626, -193.3464) knots 0 0 0 1 1 1
  spline S167 degree 2 poles (-3.9626, -193.3464) (-3.8844, -193.6121) (-3.8532, -193.698) (-3.7907, -193.7449) knots 0 0 0 1 2 2 2
  spline S168 degree 2 poles (-3.7907, -193.7449) (-3.6891, -193.8386) (-3.4548, -193.8386) knots 0 0 0 1 1 1
  line L116 (-3.4548, -193.8386) -> (3.139, -193.8386)
  spline S169 degree 2 poles (3.139, -193.8386) (3.3734, -193.8386) (3.4749, -193.7449) knots 0 0 0 1 1 1
  spline S170 degree 2 poles (3.4749, -193.7449) (3.5374, -193.698) (3.5687, -193.6121) (3.639, -193.3464) knots 0 0 0 1 2 2 2
  spline S171 degree 2 poles (3.639, -193.3464) (3.7249, -193.0339) (3.9984, -193.0339) knots 0 0 0 1 1 1
  spline S172 degree 2 poles (3.9984, -193.0339) (4.1624, -193.0339) (4.3421, -193.3386) (4.3421, -193.6277) knots 0 0 0 1 2 2 2
  line L117 (4.3421, -193.6277) -> (4.3421, -193.8308)
  line L118 (4.3421, -193.8308) -> (4.3421, -197.3542)
  line L119 (4.3421, -197.3542) -> (4.3421, -197.5574)
  spline S173 degree 2 poles (4.3421, -197.5574) (4.3421, -198.1199) (3.9984, -198.1199) knots 0 0 0 1 1 1
  spline S174 degree 2 poles (3.9984, -198.1199) (3.7249, -198.1199) (3.639, -197.823) knots 0 0 0 1 1 1
  line L120 (3.639, -197.823) -> (3.5765, -197.573)
  spline S175 degree 2 poles (3.5765, -197.573) (3.514, -197.3464) (3.139, -197.3464) knots 0 0 0 1 1 1
  line L121 (3.139, -197.3464) -> (-3.4548, -197.3464)
  spline S176 degree 2 poles (-3.4548, -197.3464) (-3.8298, -197.3464) (-3.8923, -197.573) knots 0 0 0 1 1 1
  line L122 (-3.8923, -197.573) -> (-3.9626, -197.823)
  spline S177 degree 2 poles (-3.9626, -197.823) (-4.0407, -198.1199) (-4.3141, -198.1199) knots 0 0 0 1 1 1
  spline S178 degree 2 poles (-4.3141, -198.1199) (-4.6579, -198.1199) (-4.6579, -197.5574) knots 0 0 0 1 1 1
  line L123 (-4.6579, -197.5574) -> (-4.6579, -197.3542)
  line L124 (4.3421, -209.5652) -> (-1.7516, -213.7683)
  line L125 (-1.7516, -213.7683) -> (-4.6579, -213.7683)
  line L126 (-4.6579, -213.7683) -> (-4.6579, -211.6121)
  line L127 (-4.6579, -211.6121) -> (3.0531, -206.2449)
  spline S179 degree 2 poles (3.0531, -206.2449) (3.3109, -206.0652) (3.5062, -205.8464) (3.5531, -205.6746) knots 0 0 0 1 2 2 2
  line L128 (3.5531, -205.6746) -> (3.6468, -205.3699)
  spline S180 degree 2 poles (3.6468, -205.3699) (3.6781, -205.2527) (3.8499, -205.1121) (3.9515, -205.1121) knots 0 0 0 1 2 2 2
  spline S181 degree 2 poles (3.9515, -205.1121) (4.0687, -205.1121) (4.2562, -205.2527) (4.2952, -205.3699) knots 0 0 0 1 2 2 2
  spline S182 degree 2 poles (4.2952, -205.3699) (4.3421, -205.5027) (4.3421, -206.0964) knots 0 0 0 1 1 1
  line L129 (4.3421, -206.0964) -> (4.3421, -209.5652)
  line L130 (2.0218, -206.2527) -> (0.8656, -207.0886)
  line L131 (0.8656, -207.0886) -> (-2.6657, -207.0886)
  spline S183 degree 2 poles (-2.6657, -207.0886) (-3.1266, -207.0886) (-3.7204, -207.4636) (-3.9157, -207.8621) knots 0 0 0 1 2 2 2
  line L132 (-3.9157, -207.8621) -> (-4.0251, -208.1042)
  spline S184 degree 2 poles (-4.0251, -208.1042) (-4.1266, -208.3074) (-4.3219, -208.3074) knots 0 0 0 1 1 1
  spline S185 degree 2 poles (-4.3219, -208.3074) (-4.4704, -208.3074) (-4.5719, -208.1589) knots 0 0 0 1 1 1
  spline S186 degree 2 poles (-4.5719, -208.1589) (-4.6579, -208.0339) (-4.6579, -207.6355) knots 0 0 0 1 1 1
  line L133 (-4.6579, -207.6355) -> (-4.6579, -205.8074)
  spline S187 degree 2 poles (-4.6579, -205.8074) (-4.6579, -205.0886) (-4.3141, -205.0886) knots 0 0 0 1 1 1
  spline S188 degree 2 poles (-4.3141, -205.0886) (-4.1969, -205.0886) (-4.0563, -205.2371) (-3.9391, -205.4949) knots 0 0 0 1 2 2 2
  spline S189 degree 2 poles (-3.9391, -205.4949) (-3.5876, -206.2527) (-2.6657, -206.2527) knots 0 0 0 1 1 1
  line L134 (-2.6657, -206.2527) -> (2.0218, -206.2527)
  line L135 (-0.6969, -213.7683) -> (0.4827, -212.9324)
  line L136 (0.4827, -212.9324) -> (2.3109, -212.9324)
  spline S190 degree 2 poles (2.3109, -212.9324) (2.8656, -212.9324) (3.4515, -212.5417) (3.6624, -212.0574) knots 0 0 0 1 2 2 2
  spline S191 degree 2 poles (3.6624, -212.0574) (3.7249, -211.8855) (3.8812, -211.7605) (3.9984, -211.7605) knots 0 0 0 1 2 2 2
  spline S192 degree 2 poles (3.9984, -211.7605) (4.1781, -211.7605) (4.3421, -212.0417) (4.3421, -212.3464) knots 0 0 0 1 2 2 2
  line L137 (4.3421, -212.3464) -> (4.3421, -214.323)
  spline S193 degree 2 poles (4.3421, -214.323) (4.3421, -214.7292) (4.2327, -214.8542) knots 0 0 0 1 1 1
  spline S194 degree 2 poles (4.2327, -214.8542) (4.1312, -214.9871) (3.9827, -214.9871) knots 0 0 0 1 1 1
  spline S195 degree 2 poles (3.9827, -214.9871) (3.8499, -214.9871) (3.7093, -214.8386) (3.5921, -214.5496) knots 0 0 0 1 2 2 2
  spline S196 degree 2 poles (3.5921, -214.5496) (3.4124, -214.1355) (3.0452, -213.9167) knots 0 0 0 1 1 1
  spline S197 degree 2 poles (3.0452, -213.9167) (2.7718, -213.7683) (2.3109, -213.7683) knots 0 0 0 1 1 1
  line L138 (2.3109, -213.7683) -> (-0.6969, -213.7683)
  line L139 (4.3421, -220.2761) -> (-4.6579, -220.2761)
  line L140 (-4.6579, -220.2761) -> (-4.6579, -216.7605)
  line L141 (-4.6579, -216.7605) -> (-4.6579, -216.5574)
  spline S198 degree 2 poles (-4.6579, -216.5574) (-4.6579, -216.2683) (-4.4782, -215.9636) (-4.3141, -215.9636) knots 0 0 0 1 2 2 2
  spline S199 degree 2 poles (-4.3141, -215.9636) (-4.0485, -215.9636) (-3.9626, -216.2761) knots 0 0 0 1 1 1
  spline S200 degree 2 poles (-3.9626, -216.2761) (-3.8844, -216.5417) (-3.8532, -216.6277) (-3.7907, -216.6746) knots 0 0 0 1 2 2 2
  spline S201 degree 2 poles (-3.7907, -216.6746) (-3.6891, -216.7683) (-3.4548, -216.7683) knots 0 0 0 1 1 1
  line L142 (-3.4548, -216.7683) -> (3.139, -216.7683)
  spline S202 degree 2 poles (3.139, -216.7683) (3.3734, -216.7683) (3.4749, -216.6746) knots 0 0 0 1 1 1
  spline S203 degree 2 poles (3.4749, -216.6746) (3.5374, -216.6277) (3.5687, -216.5417) (3.639, -216.2761) knots 0 0 0 1 2 2 2
  spline S204 degree 2 poles (3.639, -216.2761) (3.7249, -215.9636) (3.9984, -215.9636) knots 0 0 0 1 1 1
  spline S205 degree 2 poles (3.9984, -215.9636) (4.1624, -215.9636) (4.3421, -216.2683) (4.3421, -216.5574) knots 0 0 0 1 2 2 2
  line L143 (4.3421, -216.5574) -> (4.3421, -216.7605)
  line L144 (4.3421, -216.7605) -> (4.3421, -220.2761)
  line L145 (-4.6579, -220.9949) -> (-3.9469, -220.9949)
  spline S206 degree 2 poles (-3.9469, -220.9949) (-3.8844, -221.5105) (-3.6423, -222.1824) (-3.4001, -222.5183) knots 0 0 0 1 2 2 2
  spline S207 degree 2 poles (-3.4001, -222.5183) (-3.1579, -222.8621) (-2.6344, -223.2605) (-2.2048, -223.448) knots 0 0 0 1 2 2 2
  spline S208 degree 2 poles (-2.2048, -223.448) (-1.9938, -223.5339) (-1.8454, -223.7214) (-1.8454, -223.8855) knots 0 0 0 1 2 2 2
  spline S209 degree 2 poles (-1.8454, -223.8855) (-1.8454, -224.1121) (-2.0641, -224.2839) (-2.3298, -224.2839) knots 0 0 0 1 2 2 2
  line L146 (-2.3298, -224.2839) -> (-4.6579, -224.2839)
  line L147 (-4.6579, -224.2839) -> (-4.6579, -220.9949)
  line L148 (4.3421, -220.9871) -> (4.3421, -224.1746)
  line L149 (4.3421, -224.1746) -> (2.0062, -224.1746)
  spline S210 degree 2 poles (2.0062, -224.1746) (1.8031, -224.1746) (1.6234, -223.9871) (1.6234, -223.7761) knots 0 0 0 1 2 2 2
  spline S211 degree 2 poles (1.6234, -223.7761) (1.6234, -223.6042) (1.7406, -223.448) (1.9281, -223.3777) knots 0 0 0 1 2 2 2
  spline S212 degree 2 poles (1.9281, -223.3777) (2.6859, -223.073) (3.4906, -221.9089) (3.5687, -220.9871) knots 0 0 0 1 2 2 2
  line L150 (3.5687, -220.9871) -> (4.3421, -220.9871)
  line L151 (-0.4626, -220.948) -> (0.3031, -220.948)
  spline S213 degree 2 poles (0.3031, -220.948) (0.4906, -221.4089) (0.9281, -221.8464) (1.2874, -221.9558) knots 0 0 0 1 2 2 2
  spline S214 degree 2 poles (1.2874, -221.9558) (1.5374, -222.0183) (1.7327, -222.2214) (1.7327, -222.4089) knots 0 0 0 1 2 2 2
  spline S215 degree 2 poles (1.7327, -222.4089) (1.7327, -222.6667) (1.5687, -222.7605) knots 0 0 0 1 1 1
  spline S216 degree 2 poles (1.5687, -222.7605) (1.4827, -222.8152) (1.1781, -222.8152) knots 0 0 0 1 1 1
  line L152 (1.1781, -222.8152) -> (-1.3376, -222.8152)
  spline S217 degree 2 poles (-1.3376, -222.8152) (-1.6501, -222.8152) (-1.8844, -222.6511) (-1.8844, -222.4246) knots 0 0 0 1 2 2 2
  spline S218 degree 2 poles (-1.8844, -222.4246) (-1.8844, -222.2449) (-1.6969, -222.0417) (-1.4782, -221.9792) knots 0 0 0 1 2 2 2
  spline S219 degree 2 poles (-1.4782, -221.9792) (-1.0251, -221.8386) (-0.5407, -221.3464) (-0.4626, -220.948) knots 0 0 0 1 2 2 2
  line L153 (4.3421, -229.7839) -> (-3.4079, -229.7839)
  spline S220 degree 2 poles (-3.4079, -229.7839) (-3.6657, -229.7839) (-3.7751, -229.9011) knots 0 0 0 1 1 1
  spline S221 degree 2 poles (-3.7751, -229.9011) (-3.8376, -229.9636) (-3.8766, -230.0808) (-3.9391, -230.3855) knots 0 0 0 1 2 2 2
  spline S222 degree 2 poles (-3.9391, -230.3855) (-4.0094, -230.7683) (-4.2985, -230.7683) knots 0 0 0 1 1 1
  spline S223 degree 2 poles (-4.2985, -230.7683) (-4.4704, -230.7683) (-4.5798, -230.5652) knots 0 0 0 1 1 1
  spline S224 degree 2 poles (-4.5798, -230.5652) (-4.6579, -230.4089) (-4.6579, -230.0652) knots 0 0 0 1 1 1
  line L154 (-4.6579, -230.0652) -> (-4.6579, -229.7917)
  line L155 (-4.6579, -229.7917) -> (-4.6579, -226.2683)
  line L156 (-4.6579, -226.2683) -> (-4.6579, -226.0652)
  spline S225 degree 2 poles (-4.6579, -226.0652) (-4.6579, -225.7761) (-4.4782, -225.4714) (-4.3141, -225.4714) knots 0 0 0 1 2 2 2
  spline S226 degree 2 poles (-4.3141, -225.4714) (-4.0485, -225.4714) (-3.9626, -225.7839) knots 0 0 0 1 1 1
  spline S227 degree 2 poles (-3.9626, -225.7839) (-3.8844, -226.0496) (-3.8532, -226.1355) (-3.7907, -226.1824) knots 0 0 0 1 2 2 2
  spline S228 degree 2 poles (-3.7907, -226.1824) (-3.6891, -226.2761) (-3.4548, -226.2761) knots 0 0 0 1 1 1
  line L157 (-3.4548, -226.2761) -> (3.139, -226.2761)
  spline S229 degree 2 poles (3.139, -226.2761) (3.3734, -226.2761) (3.4749, -226.1824) knots 0 0 0 1 1 1
  spline S230 degree 2 poles (3.4749, -226.1824) (3.5374, -226.1355) (3.5687, -226.0496) (3.639, -225.7839) knots 0 0 0 1 2 2 2
  spline S231 degree 2 poles (3.639, -225.7839) (3.7249, -225.4714) (3.9984, -225.4714) knots 0 0 0 1 1 1
  spline S232 degree 2 poles (3.9984, -225.4714) (4.1624, -225.4714) (4.3421, -225.7761) (4.3421, -226.0652) knots 0 0 0 1 2 2 2
  line L158 (4.3421, -226.0652) -> (4.3421, -226.2683)
  line L159 (4.3421, -226.2683) -> (4.3421, -229.7839)
  spline S233 degree 2 poles (-0.2516, -232.2136) (-0.3376, -232.9402) (-0.5641, -233.7292) (-0.7594, -234.0417) knots 0 0 0 1 2 2 2
  spline S234 degree 2 poles (-0.7594, -234.0417) (-0.9626, -234.3699) (-1.5251, -234.7292) (-1.8454, -234.7292) knots 0 0 0 1 2 2 2
  line L160 (-1.8454, -234.7292) -> (-3.2048, -234.7292)
  spline S235 degree 2 poles (-3.2048, -234.7292) (-3.4235, -234.7292) (-3.4235, -234.8933) knots 0 0 0 1 1 1
  spline S236 degree 2 poles (-3.4235, -234.8933) (-3.4235, -234.9558) (-3.361, -235.0496) (-3.2751, -235.1277) knots 0 0 0 1 2 2 2
  spline S237 degree 2 poles (-3.2751, -235.1277) (-3.0485, -235.323) (-3.0485, -235.5261) knots 0 0 0 1 1 1
  spline S238 degree 2 poles (-3.0485, -235.5261) (-3.0485, -235.6667) (-3.2829, -235.9324) (-3.4079, -235.9324) knots 0 0 0 1 2 2 2
  spline S239 degree 2 poles (-3.4079, -235.9324) (-3.611, -235.9324) (-4.1969, -235.4636) (-4.4313, -235.1199) knots 0 0 0 1 2 2 2
  spline S240 degree 2 poles (-4.4313, -235.1199) (-4.6423, -234.7917) (-4.8376, -234.0339) (-4.8376, -233.5183) knots 0 0 0 1 2 2 2
  spline S241 degree 2 poles (-4.8376, -233.5183) (-4.8376, -232.4792) (-3.8376, -231.3074) (-2.9548, -231.3074) knots 0 0 0 1 2 2 2
  line L161 (-2.9548, -231.3074) -> (-1.8454, -231.3074)
  spline S242 degree 2 poles (-1.8454, -231.3074) (-1.4782, -231.3074) (-1.4157, -231.2996) knots 0 0 0 1 1 1
  spline S243 degree 2 poles (-1.4157, -231.2996) (-1.1501, -231.2605) (-0.9626, -231.0808) knots 0 0 0 1 1 1
  spline S244 degree 2 poles (-0.9626, -231.0808) (-0.7282, -230.8464) (-0.6891, -230.4246) knots 0 0 0 1 1 1
  line L162 (-0.6891, -230.4246) -> (0.014, -230.4246)
  spline S245 degree 2 poles (0.014, -230.4246) (0.0687, -230.8464) (0.2015, -231.0339) knots 0 0 0 1 1 1
  spline S246 degree 2 poles (0.2015, -231.0339) (0.3187, -231.1902) (0.6234, -231.3074) (0.9202, -231.3074) knots 0 0 0 1 2 2 2
  line L163 (0.9202, -231.3074) -> (2.6702, -231.3074)
  spline S247 degree 2 poles (2.6702, -231.3074) (3.0843, -231.3074) (3.4906, -230.9167) (3.6077, -230.4167) knots 0 0 0 1 2 2 2
  line L164 (3.6077, -230.4167) -> (4.3421, -230.4167)
  line L165 (4.3421, -230.4167) -> (4.3421, -230.6199)
  spline S248 degree 2 poles (4.3421, -230.6199) (4.3421, -231.4949) (4.2874, -232.1121) knots 0 0 0 1 1 1
  spline S249 degree 2 poles (4.2874, -232.1121) (4.2171, -233.0261) (3.7874, -233.7449) knots 0 0 0 1 1 1
  spline S250 degree 2 poles (3.7874, -233.7449) (3.1781, -234.7839) (2.0374, -234.7839) knots 0 0 0 1 1 1
  spline S251 degree 2 poles (2.0374, -234.7839) (1.1077, -234.7839) (0.514, -234.0886) knots 0 0 0 1 1 1
  spline S252 degree 2 poles (0.514, -234.0886) (0.264, -233.7996) (-0.0485, -233.0105) (-0.2516, -232.2136) knots 0 0 0 1 2 2 2
  point P0 (0, 0)
  constraints: 2 other
extrude "Extrusion3" cut sketch "Skizze8" against normal blind 10 contours L13 L14 L15 S0 S1 S2 S3 L16 S4 S5 S6 S7 L17 L18 | L19 S8 S9 S10 S11 L20 L21 | L22 L23 S12 S13 S14 L24 | L25 S15 S16 S17 S18 L26 S19 S20 S21 | L27 L28 S22 S23 S24 S25 L29 S26 S27 S28 S29 L30 L31 L32 S30 S31 S32 S33 L33 S34 S35 S36 S37 L34 | L35 S38 S39 S40 S41 S42 S43 S44 L36 S45 S46 S47 S48 S49 S50 S51 | L37 S52 S53 S54 S55 S56 L38 S57 S58 S59 S60 | L39 S61 S62 S63 L40 S64 S65 L41 S66 S67 S68 S69 S70 | L42 L43 L44 S71 S72 S73 S74 L45 S75 S76 S77 S78 L46 L47 | L48 S79 S80 S81 S82 L49 L50 | L51 L52 S83 S84 S85 L53 | L54 S86 S87 S88 S89 L55 S90 S91 S92 | L56 L57 L58 L59 S93 L60 S94 S95 S96 L61 | L62 L63 S97 L64 S98 S99 S100 L65 S101 S102 S103 L66 | L67 L68 S104 S105 S106 L69 S107 S108 S109 S110 S111 L70 | L71 L72 L73 S112 S113 S114 S115 L74 S116 S117 S118 S119 L75 L76 | S120 S121 S122 S123 L77 L78 S124 S125 L79 S126 S127 L80 S128 S129 L81 L82 S130 S131 L83 L84 S132 S133 S134 S135 | L85 L86 S136 S137 S138 S139 L87 S140 S141 S142 S143 L88 L89 L90 L91 L92 L93 | L94 L95 S144 S145 L96 S146 S147 L97 S148 S149 S150 S151 L98 | L99 L100 S152 L101 S153 S154 L102 L103 L104 S155 S156 S157 S158 L105 S159 L106 S160 S161 L107 L108 L109 S162 S163 L110 S164 L111 L112 L113 | L114 L115 S165 S166 S167 S168 L116 S169 S170 S171 S172 L117 L118 L119 S173 S174 L120 S175 L121 S176 L122 S177 S178 L123 | L124 L125 L126 L127 S179 L128 S180 S181 S182 L129 | L130 L131 S183 L132 S184 S185 S186 L133 S187 S188 S189 L134 | L135 L136 S190 S191 S192 L137 S193 S194 S195 S196 S197 L138 | L139 L140 L141 S198 S199 S200 S201 L142 S202 S203 S204 S205 L143 L144 | L145 S206 S207 S208 S209 L146 L147 | L148 L149 S210 S211 S212 L150 | L151 S213 S214 S215 S216 L152 S217 S218 S219 | L153 S220 S221 S222 S223 S224 L154 L155 L156 S225 S226 S227 S228 L157 S229 S230 S231 S232 L158 L159 | S233 S234 L160 S235 S236 S237 S238 S239 S240 S241 L161 S242 S243 S244 L162 S245 S246 L163 S247 L164 L165 S248 S249 S250 S251 S252
equation "\"d125\" = Stärke"
equation "\"d6\" = Stärke"
equation "\"d7\" = BreiteBiegungsfreistellung"
equation "\"d8\" = TiefeBiegungsfreistellung"
equation "\"d9\" = MinimalRest"
equation "\"d10\" = Übergangsradius"
equation "\"d13\" = Biegeradius"
equation "\"d14\" = GrößeEckenfreistellung"
equation "\"d15\" = Abstandsgröße"
equation "\"d16\" = JacobiRadiusGröße"
equation "\"d17\" = BreiteBiegungsfreistellung"
equation "\"d18\" = TiefeBiegungsfreistellung"
equation "\"d19\" = MinimalRest"
equation "\"d20\" = Übergangsradius"
equation "\"d23\" = Biegeradius"
equation "\"d24\" = GrößeEckenfreistellung"
equation "\"d25\" = Abstandsgröße"
equation "\"d26\" = JacobiRadiusGröße"
equation "\"Biegeradius\" = Stärke"
equation "\"BreiteBiegungsfreistellung\" = Stärke"
equation "\"TiefeBiegungsfreistellung\" = 0.5 * Stärke"
equation "\"GrößeEckenfreistellung\" = 4 * Stärke"
equation "\"MinimalRest\" = 2 * Stärke"
equation "\"Übergangsradius\" = Biegeradius"
equation "\"JacobiRadiusGröße\" = Biegeradius"
equation "\"Abstandsgröße\" = Stärke"
equation "\"Stärke\" = 2"
